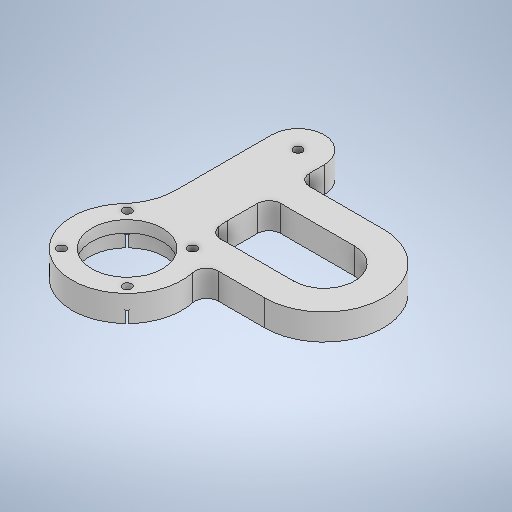
# Autodesk Inventor part: leg_extend_R
Saved by Autodesk Inventor 2025.2 (Build 292293000, 293)
## iProperties
Created: 2025-04-10
Part Number: leg_extend_R
Material: Generic
Document SubType Name: Modeling
Designer: Bruno
Density: 1 g/cm^3
Appearance: Default
Author: Bruno
## iProperties of the stored document leg_extend_3DPrint.ipt
Created: 2025-04-23
Part Number: leg_extend_3DPrint
Material: Generic
Document SubType Name: Modeling
Designer: Bruno
Density: 1 g/cm^3
Appearance: Default
Author: Bruno
Autodesk Inventor part; units mm, degrees
ref_plane "YZ Plane" through (0, 0, 0) normal (1, 0, 0) x (0, 1, 0)
ref_plane "XZ Plane" through (0, 0, 0) normal (0, 1, 0) x (-1, 0, 0)
ref_plane "XY Plane" through (0, 0, 0) normal (0, 0, 1) x (1, 0, 0)
sketch "Sketch1" plane through (0, 0, 0) normal (0, 1, 0) x (-1, 0, 0)
  line L0 (0, -55.9) -> (0, 65.9) construction
  line L1 (0, 29.5) -> (0, -29.5) construction
  arc A0 (14, 16.6548) -> (-14, 16.6548) centre (0, 29.5) ccw
  arc A1 (-9, -29.5) -> (9, -29.5) centre (0, -29.5) ccw
  line L2 (9, -29.5) -> (9, 3.8095)
  arc A2 (14, 16.6548) -> (9, 3.8095) centre (28, 3.8095) ccw
  line L3 (-9, -29.5) -> (-9, 3.8095)
  arc A3 (-9, 3.8095) -> (-14, 16.6548) centre (-28, 3.8095) ccw
  circle A4 centre (0, 29.5) radius 13.0325
  circle A5 centre (-38.5, 0) radius 10.5
  arc A6 (-38.5, 20.5) -> (-38.5, -20.5) centre (-38.5, 0) ccw
  line L4 (-38.5, 20.5) -> (-16.7332, 20.5)
  line L5 (-38.5, -20.5) -> (-9, -20.5)
  line L6 (-38.5, -10.5) -> (-9, -10.5)
  line L7 (-38.5, 10.5) -> (-10.2169, 10.5)
  point P0 (0, 0)
  point P1 (0, 0)
  point P2 (0, -38.5)
  point P3 (-5.5975, 47.6568)
  point P4 (-18.642, 33.1709)
  point P5 (-35.056, 9.9191)
  point P6 (-9, -28.5)
  point P7 (-59, 0)
  dimension "d0" = 59
  dimension "d1" = 29.5
  dimension "d2" = 38
  dimension "d3" = 18
  dimension "d4" = 19
  dimension "d5" = 26.065
  dimension "d31" = 10
  dimension "d32" = 59
  constraints: 19 point on circle, 14 end point, 8 tangent, 7 centre point, 5 point on line, 4 coincident, 4 horizontal, 4 symmetric about line, 1 horizontal alignment, 1 midpoint, 1 vertical, 1 other
  measures "d0" distance of L1.start L1.end
  measures "d1" distance of L1.end point (0, 0)
  measures "d2" diameter of A0
  measures "d3" diameter of A1
  measures "d4" radius of A2
  measures "d5" diameter of A4
  measures "d31" radial gap between concentric circles of A5 A6
  measures "d32" distance of point (0, 0) point (-59, 0)
extrude "Extrusion1" add sketch "Sketch1" along normal blind 9 contours A2 L2 A1 L3 A3 A0 | A0 A3 L7 A5 L6 L3 L5 A6 L4
sketch "Sketch2" plane through (0, 0, 0) normal (0, -1, 0) x (1, 0, 0)
  circle A0 centre (0, 29.5) radius 13.0325 projected
  circle A1 centre (0, 29.5) radius 12.1825
  point P0 (0, 0)
  dimension "d8" = 0.85
  constraints: 1 centre point, 1 coincident
  measures "d8" radial gap between concentric circles of A0 A1
extrude "Extrusion2" add sketch "Sketch2" against normal blind 4
sketch "Sketch3" plane through (0, 9, 0) normal (0, 1, 0) x (1, 0, 0)
  arc A0 (9, 29.5) -> (-9, 29.5) centre (0, 29.5) ccw projected
  circle A1 centre (0, 29.5) radius 1.5
  point P0 (0, 0)
  point P1 (0, 38.5)
  dimension "d11" = 3
  constraints: 1 centre point, 1 coincident
  measures "d11" diameter of A1
extrude "Extrusion3" cut sketch "Sketch3" against normal through all
sketch "Sketch4" plane through (0, 9, 0) normal (0, 1, 0) x (1, 0, 0)
  circle A0 centre (0, -29.5) radius 12.1825 projected
  line L0 (0, -29.5) -> (0, -21.0642) construction
  circle A1 centre (0, -29.5) radius 16.0162 construction
  circle A2 centre (0, -29.5) radius 13.0325 projected
  line L1 (-13.0325, -29.5) -> (-16.0162, -29.5) construction
  line L2 (-16.0162, -29.5) -> (-19, -29.5) construction
  arc A3 (-14, -16.6548) -> (16.7332, -20.5) centre (0, -29.5) ccw projected
  line L3 (0, -29.5) -> (-11.3252, -18.1748) construction
  circle A4 centre (-11.3252, -18.1748) radius 1.5
  circle A5 centre (-11.3252, -40.8252) radius 1.5
  circle A6 centre (11.3252, -40.8252) radius 1.5
  circle A7 centre (11.3252, -18.1748) radius 1.5
  point P0 (0, 0)
  point P1 (14, -16.6548)
  dimension "d14" = 45
  dimension "d15" = 3
  dimension "d18" = 360
  constraints: 8 end point, 5 centre point, 3 point on circle, 2 coincident, 2 horizontal, 1 collinear, 1 horizontal alignment, 1 point on line, 1 vertical, 10 other
  measures "d14" angle of L3 L0
  measures "d15" diameter of A4
extrude "Extrusion4" cut sketch "Sketch4" against normal through all contours A4 | A5 | A6 | A7
sketch "Sketch5" plane through (0, 9, 0) normal (0, 1, 0) x (1, 0, 0)
  circle A0 centre (-11.3252, -40.8252) radius 1.5 projected
  circle A1 centre (-11.3252, -40.8252) radius 3
  circle A2 centre (-11.3252, -18.1748) radius 1.5 projected
  circle A3 centre (-11.3252, -18.1748) radius 3
  circle A4 centre (11.3252, -40.8252) radius 1.5 projected
  circle A5 centre (11.3252, -40.8252) radius 3
  circle A6 centre (11.3252, -18.1748) radius 1.5 projected
  circle A7 centre (11.3252, -18.1748) radius 3
  point P0 (0, 0)
  dimension "d22" = 6
  dimension "d23" = 6
  dimension "d24" = 6
  dimension "d25" = 6
  constraints: 4 centre point, 4 coincident
  measures "d22" diameter of A1
  measures "d23" diameter of A3
  measures "d24" diameter of A5
  measures "d25" diameter of A7
extrude "Extrusion5" cut sketch "Sketch5" against normal blind 4 contours A0 | A1 | A2 | A3 | A4 | A5 | A6 | A7
fillet "Fillet2" radius 4 4 edges at (16.7332, 4.5, 20.5) (10.2169, 4.5, 10.5) (9, 4.5, -10.5) (9, 4.5, -20.5)
mirror "Mirror1" about plane through (0, 0, 0) normal (0, 1, 0) remove original yes
equation "\"d1\" = 0.5 * d0"
equation "\"d4\" = 0.5 * d2"
body "Solid1"
